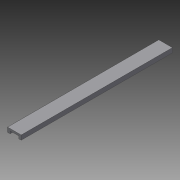
# Autodesk Inventor part: profilo_estrusore
Saved by Autodesk Inventor 2014 SP1 (Build 180222100, 222)
## iProperties
Created: 2015-04-15
Part Number: profilo_estrusore
Material: Generic
Document SubType Name: Modeling
Designer: Giorgio Nuzzo
Density: 1 g/cm^3
Appearance: Default
Author: Giorgio Nuzzo
Autodesk Inventor part; units mm, degrees
ref_plane "YZ Plane" through (0, 0, 0) normal (1, 0, 0) x (0, 1, 0)
ref_plane "XZ Plane" through (0, 0, 0) normal (0, 1, 0) x (-1, 0, 0)
ref_plane "XY Plane" through (0, 0, 0) normal (0, 0, 1) x (1, 0, 0)
sketch "Sketch1" plane through (0, 0, 0) normal (0, 1, 0) x (-1, 0, 0)
  line L0 (-13.5, 4.5) -> (13.5, 4.5)
  line L1 (13.5, 4.5) -> (13.5, -4.5)
  line L2 (13.5, -4.5) -> (-13.5, -4.5) construction
  line L3 (-13.5, -4.5) -> (-13.5, 4.5)
  line L4 (0, -6.3) -> (0, 6.3) construction
  line L5 (-18.9, 0) -> (18.9, 0) construction
  line L6 (-13.5, -4.5) -> (-8.5, -4.5)
  line L7 (13.5, -4.5) -> (8.5, -4.5)
  line L8 (-8.5, -4.5) -> (-8.5, 0.5)
  line L9 (-8.5, 0.5) -> (8.5, 0.5)
  line L10 (8.5, 0.5) -> (8.5, -4.5)
  point P0 (0, 0)
  dimension "d0" = 27
  dimension "d1" = 9
  dimension "d2" = 5
  dimension "d3" = 5
  dimension "d4" = 5
  constraints: 18 end point, 3 parallel, 3 perpendicular, 2 point on line, 1 horizontal, 2 other
  measures "d0" distance of L0.start L0.end
  measures "d1" distance of L2.end L0.start
  measures "d2" distance of L2.end L6.end
  measures "d3" distance of L1.end L7.end
  measures "d4" distance between parallel lines of L2 L9
extrude "Extrusion1" add sketch "Sketch1" along normal blind 300
equation "\"d3\" = d2"
body "Solid1"
